Autodesk Fusion 360 part; units mm, degrees
(part 8 of 14)
  line L3484 (76.692, 59.464) -> (76.692, 60.314)
  arc A2247 (75.7545, 60.189) -> (75.6295, 60.189) centre (75.692, 60.189) ccw
  line L3485 (77.242, 58.9765) -> (77.842, 58.9765)
  line L3486 (76.6295, 60.189) -> (76.6295, 59.589)
  line L3487 (76.192, 55.764) -> (76.192, 56.614)
  line L3488 (76.2545, 59.589) -> (76.2545, 60.189)
  line L3489 (75.7545, 59.589) -> (75.7545, 60.189)
  line L3490 (77.967, 58.039) -> (77.117, 58.039)
  line L3491 (76.692, 55.764) -> (76.692, 56.614)
  arc A2248 (75.1295, 59.589) -> (75.2545, 59.589) centre (75.192, 59.589) ccw
  line L3492 (74.692, 59.464) -> (74.692, 60.314)
  line L3493 (76.192, 59.464) -> (76.192, 60.314)
  line L3494 (76.692, 55.764) -> (76.692, 56.614)
  line L3495 (74.142, 59.1015) -> (73.542, 59.1015)
  line L3496 (74.6295, 60.189) -> (74.6295, 59.589)
  arc A2249 (76.6295, 55.889) -> (76.7545, 55.889) centre (76.692, 55.889) ccw
  line L3497 (74.267, 58.539) -> (73.417, 58.539)
  arc A2250 (73.542, 58.6015) -> (73.542, 58.4765) centre (73.542, 58.539) ccw
  arc A2251 (74.142, 57.9765) -> (74.142, 58.1015) centre (74.142, 58.039) ccw
  arc A2252 (80.495, 51.1923) -> (80.495, 51.2558) centre (80.495, 51.224) ccw
  line L3498 (73.542, 56.9765) -> (74.142, 56.9765)
  line L3499 (81.745, 51.782) -> (81.745, 51.224)
  arc A2253 (79.545, 50.9358) -> (79.545, 50.8723) centre (79.545, 50.904) ccw
  line L3500 (79.545, 50.904) -> (80.495, 50.904)
  line L3501 (74.267, 57.539) -> (73.417, 57.539)
  arc A2254 (79.545, 51.8137) -> (79.545, 51.7502) centre (79.545, 51.782) ccw
  line L3502 (79.545, 51.224) -> (79.545, 51.782)
  arc A2255 (74.142, 58.4765) -> (74.142, 58.6015) centre (74.142, 58.539) ccw
  arc A2256 (73.542, 57.6015) -> (73.542, 57.4765) centre (73.542, 57.539) ccw
  line L3503 (73.542, 57.4765) -> (74.142, 57.4765)
  line L3504 (74.142, 57.1015) -> (73.542, 57.1015)
  line L3505 (74.267, 57.039) -> (73.417, 57.039)
  arc A2257 (74.142, 57.4765) -> (74.142, 57.6015) centre (74.142, 57.539) ccw
  line L3506 (78.78, 53.054) -> (78.645, 52.919)
  line L3507 (80.785, 50.904) -> (81.745, 50.904)
  line L3508 (80.785, 51.224) -> (80.785, 52.154)
  arc A2258 (81.745, 50.2943) -> (81.745, 50.3578) centre (81.745, 50.326) ccw
  arc A2259 (80.785, 49.9223) -> (80.785, 49.9858) centre (80.785, 49.954) ccw
  line L3509 (73.542, 57.9765) -> (74.142, 57.9765)
  arc A2260 (80.495, 49.9858) -> (80.495, 49.9223) centre (80.495, 49.954) ccw
  line L3510 (80.495, 52.154) -> (80.495, 51.224)
  line L3511 (80.495, 49.954) -> (79.917, 49.954)
  line L3512 (74.142, 58.1015) -> (73.542, 58.1015)
  arc A2261 (79.545, 51.1923) -> (79.545, 51.2558) centre (79.545, 51.224) ccw
  line L3513 (79.917, 52.154) -> (80.495, 52.154)
  line L3514 (75.692, 56.964) -> (75.692, 59.114)
  line L3515 (81.373, 49.954) -> (80.785, 49.954)
  line L3516 (79.917, 49.954) -> (79.545, 50.326)
  line L3517 (81.745, 50.904) -> (81.745, 50.326)
  arc A2262 (81.373, 49.9223) -> (81.373, 49.9858) centre (81.373, 49.954) ccw
  line L3518 (81.745, 50.326) -> (81.373, 49.954)
  arc A2263 (81.745, 50.8723) -> (81.745, 50.9358) centre (81.745, 50.904) ccw
  arc A2264 (73.542, 58.1015) -> (73.542, 57.9765) centre (73.542, 58.039) ccw
  line L3519 (74.267, 58.039) -> (73.417, 58.039)
  arc A2265 (74.142, 56.9765) -> (74.142, 57.1015) centre (74.142, 57.039) ccw
  line L3520 (74.267, 57.539) -> (73.417, 57.539)
  line L3521 (75.692, 56.964) -> (75.692, 59.114)
  arc A2266 (81.745, 51.2558) -> (81.745, 51.1923) centre (81.745, 51.224) ccw
  arc A2267 (80.785, 49.9858) -> (80.785, 49.9223) centre (80.785, 49.954) ccw
  line L3522 (74.142, 57.6015) -> (73.542, 57.6015)
  line L3523 (81.62, 52.654) -> (81.62, 53.454)
  arc A2268 (80.495, 52.1857) -> (80.495, 52.1222) centre (80.495, 52.154) ccw
  line L3524 (73.542, 58.4765) -> (74.142, 58.4765)
  arc A2269 (81.373, 52.1222) -> (81.373, 52.1857) centre (81.373, 52.154) ccw
  line L3525 (74.267, 58.039) -> (73.417, 58.039)
  arc A2270 (81.745, 50.3578) -> (81.745, 50.2943) centre (81.745, 50.326) ccw
  line L3526 (74.267, 57.039) -> (73.417, 57.039)
  line L3527 (80.495, 50.904) -> (80.495, 49.954)
  arc A2271 (81.373, 52.1857) -> (81.373, 52.1222) centre (81.373, 52.154) ccw
  arc A2272 (79.545, 51.2558) -> (79.545, 51.1923) centre (79.545, 51.224) ccw
  line L3528 (79.545, 50.326) -> (79.545, 50.904)
  arc A2273 (80.785, 50.8723) -> (80.785, 50.9358) centre (80.785, 50.904) ccw
  arc A2274 (79.545, 50.8723) -> (79.545, 50.9358) centre (79.545, 50.904) ccw
  arc A2275 (76.067, 58.039) -> (75.317, 58.039) centre (75.692, 58.039) ccw
  arc A2276 (80.785, 50.9358) -> (80.785, 50.8723) centre (80.785, 50.904) ccw
  arc A2277 (81.373, 49.9858) -> (81.373, 49.9223) centre (81.373, 49.954) ccw
  arc A2278 (73.542, 57.1015) -> (73.542, 56.9765) centre (73.542, 57.039) ccw
  arc A2279 (80.495, 50.8723) -> (80.495, 50.9358) centre (80.495, 50.904) ccw
  arc A2280 (81.745, 50.9358) -> (81.745, 50.8723) centre (81.745, 50.904) ccw
  arc A2281 (75.317, 58.039) -> (76.067, 58.039) centre (75.692, 58.039) ccw
  line L3529 (80.32, 52.654) -> (80.32, 53.454)
  line L3530 (78.645, 52.919) -> (78.645, 49.189)
  line L3531 (81.745, 51.224) -> (80.785, 51.224)
  arc A2282 (80.495, 50.9358) -> (80.495, 50.8723) centre (80.495, 50.904) ccw
  line L3532 (81.62, 52.654) -> (81.62, 53.454)
  line L3533 (78.78, 49.054) -> (82.51, 49.054)
  line L3534 (79.545, 51.782) -> (79.917, 52.154)
  arc A2283 (80.495, 49.9223) -> (80.495, 49.9858) centre (80.495, 49.954) ccw
  line L3535 (79.045, 51.379) -> (78.245, 51.379)
  arc A2284 (82.13, 53.919) -> (82.13, 53.519) centre (82.13, 53.719) ccw
  line L3536 (79.045, 51.379) -> (78.245, 51.379)
  line L3537 (79.045, 52.029) -> (78.245, 52.029)
  line L3538 (79.045, 51.379) -> (78.245, 51.379)
  line L3539 (79.045, 50.079) -> (78.245, 50.079)
  arc A2285 (79.917, 52.1222) -> (79.917, 52.1857) centre (79.917, 52.154) ccw
  line L3540 (79.67, 48.654) -> (79.67, 49.454)
  arc A2286 (79.917, 52.1857) -> (79.917, 52.1222) centre (79.917, 52.154) ccw
  arc A2287 (80.495, 51.2558) -> (80.495, 51.1923) centre (80.495, 51.224) ccw
  line L3541 (80.97, 52.654) -> (80.97, 53.454)
  line L3542 (79.67, 52.654) -> (79.67, 53.454)
  arc A2288 (82.045, 52.754) -> (82.045, 52.354) centre (82.045, 52.554) ccw
  line L3543 (82.51, 53.054) -> (78.78, 53.054)
  arc A2289 (80.785, 52.1857) -> (80.785, 52.1222) centre (80.785, 52.154) ccw
  line L3544 (81.373, 52.154) -> (81.745, 51.782)
  line L3545 (79.045, 50.079) -> (78.245, 50.079)
  line L3546 (79.67, 48.654) -> (79.67, 49.454)
  line L3547 (79.045, 50.729) -> (78.245, 50.729)
  line L3548 (79.67, 52.654) -> (79.67, 53.454)
  arc A2290 (79.545, 50.2943) -> (79.545, 50.3578) centre (79.545, 50.326) ccw
  arc A2291 (79.545, 50.3578) -> (79.545, 50.2943) centre (79.545, 50.326) ccw
  arc A2292 (81.745, 51.8137) -> (81.745, 51.7502) centre (81.745, 51.782) ccw
  arc A2293 (80.785, 51.1923) -> (80.785, 51.2558) centre (80.785, 51.224) ccw
  line L3549 (82.51, 49.054) -> (82.645, 49.189)
  line L3550 (80.97, 48.654) -> (80.97, 49.454)
  arc A2294 (82.13, 53.519) -> (82.13, 53.919) centre (82.13, 53.719) ccw
  line L3551 (79.045, 52.029) -> (78.245, 52.029)
  line L3552 (79.045, 52.029) -> (78.245, 52.029)
  arc A2295 (81.745, 51.1923) -> (81.745, 51.2558) centre (81.745, 51.224) ccw
  line L3553 (81.62, 52.654) -> (81.62, 53.454)
  line L3554 (80.97, 52.654) -> (80.97, 53.454)
  arc A2296 (79.917, 49.9858) -> (79.917, 49.9223) centre (79.917, 49.954) ccw
  line L3555 (80.32, 52.654) -> (80.32, 53.454)
  line L3556 (80.32, 52.654) -> (80.32, 53.454)
  arc A2297 (80.495, 52.1222) -> (80.495, 52.1857) centre (80.495, 52.154) ccw
  arc A2298 (82.045, 52.354) -> (82.045, 52.754) centre (82.045, 52.554) ccw
  line L3557 (82.645, 49.189) -> (82.645, 52.919)
  line L3558 (82.645, 52.919) -> (82.51, 53.054)
  line L3559 (78.645, 49.189) -> (78.78, 49.054)
  line L3560 (79.045, 50.079) -> (78.245, 50.079)
  line L3561 (79.045, 50.729) -> (78.245, 50.729)
  arc A2299 (80.785, 51.2558) -> (80.785, 51.1923) centre (80.785, 51.224) ccw
  line L3562 (80.495, 51.224) -> (79.545, 51.224)
  line L3563 (80.785, 52.154) -> (81.373, 52.154)
  arc A2300 (79.917, 49.9223) -> (79.917, 49.9858) centre (79.917, 49.954) ccw
  line L3564 (79.67, 48.654) -> (79.67, 49.454)
  line L3565 (80.32, 48.654) -> (80.32, 49.454)
  arc A2301 (80.785, 52.1222) -> (80.785, 52.1857) centre (80.785, 52.154) ccw
  arc A2302 (81.745, 51.7502) -> (81.745, 51.8137) centre (81.745, 51.782) ccw
  line L3566 (79.67, 52.654) -> (79.67, 53.454)
  line L3567 (80.97, 52.654) -> (80.97, 53.454)
  line L3568 (80.32, 48.654) -> (80.32, 49.454)
  line L3569 (80.97, 48.654) -> (80.97, 49.454)
  arc A2303 (79.545, 51.7502) -> (79.545, 51.8137) centre (79.545, 51.782) ccw
  line L3570 (80.32, 48.654) -> (80.32, 49.454)
  line L3571 (25.865, 33.063) -> (24.905, 33.063)
  line L3572 (24.905, 33.993) -> (25.493, 33.993)
  arc A2304 (25.493, 34.0247) -> (25.493, 33.9612) centre (25.493, 33.993) ccw
  arc A2305 (24.615, 32.7748) -> (24.615, 32.7113) centre (24.615, 32.743) ccw
  line L3573 (24.615, 33.993) -> (24.615, 33.063)
  arc A2306 (25.865, 33.5892) -> (25.865, 33.6527) centre (25.865, 33.621) ccw
  line L3574 (24.905, 31.793) -> (24.905, 32.743)
  line L3575 (80.6392, 49.71) -> (80.6392, 52.41)
  line L3576 (81.62, 48.654) -> (81.62, 49.454)
  line L3577 (24.615, 31.793) -> (24.037, 31.793)
  arc A2307 (24.615, 31.8248) -> (24.615, 31.7613) centre (24.615, 31.793) ccw
  line L3578 (26.63, 30.893) -> (26.765, 31.028)
  line L3579 (79.045, 50.729) -> (78.245, 50.729)
  line L3580 (25.493, 31.793) -> (24.905, 31.793)
  line L3581 (22.9, 30.893) -> (26.63, 30.893)
  arc A2308 (25.865, 32.7748) -> (25.865, 32.7113) centre (25.865, 32.743) ccw
  line L3582 (83.045, 52.029) -> (82.245, 52.029)
  line L3583 (83.045, 50.079) -> (82.245, 50.079)
  line L3584 (83.045, 51.379) -> (82.245, 51.379)
  line L3585 (83.045, 51.379) -> (82.245, 51.379)
  line L3586 (24.905, 32.743) -> (25.865, 32.743)
  arc A2309 (24.905, 31.8248) -> (24.905, 31.7613) centre (24.905, 31.793) ccw
  line L3587 (24.037, 31.793) -> (23.665, 32.165)
  arc A2310 (24.905, 31.7613) -> (24.905, 31.8248) centre (24.905, 31.793) ccw
  arc A2311 (24.037, 31.8248) -> (24.037, 31.7613) centre (24.037, 31.793) ccw
  line L3588 (25.493, 33.993) -> (25.865, 33.621)
  arc A2312 (24.037, 31.7613) -> (24.037, 31.8248) centre (24.037, 31.793) ccw
  line L3589 (23.665, 33.621) -> (24.037, 33.993)
  arc A2313 (24.615, 31.7613) -> (24.615, 31.8248) centre (24.615, 31.793) ccw
  arc A2314 (24.615, 34.0247) -> (24.615, 33.9612) centre (24.615, 33.993) ccw
  arc A2315 (23.665, 33.0948) -> (23.665, 33.0313) centre (23.665, 33.063) ccw
  arc A2316 (25.865, 32.1333) -> (25.865, 32.1968) centre (25.865, 32.165) ccw
  line L3590 (83.045, 52.029) -> (82.245, 52.029)
  line L3591 (26.63, 34.893) -> (22.9, 34.893)
  arc A2317 (25.493, 31.8248) -> (25.493, 31.7613) centre (25.493, 31.793) ccw
  line L3592 (22.765, 34.758) -> (22.765, 31.028)
  arc A2318 (23.665, 32.1333) -> (23.665, 32.1968) centre (23.665, 32.165) ccw
  line L3593 (83.045, 50.729) -> (82.245, 50.729)
  line L3594 (23.665, 33.063) -> (23.665, 33.621)
  arc A2319 (25.493, 31.7613) -> (25.493, 31.8248) centre (25.493, 31.793) ccw
  line L3595 (25.865, 32.743) -> (25.865, 32.165)
  line L3596 (83.045, 52.029) -> (82.245, 52.029)
  line L3597 (83.045, 50.079) -> (82.245, 50.079)
  line L3598 (80.6392, 49.71) -> (80.6392, 52.41)
  line L3599 (25.865, 32.165) -> (25.493, 31.793)
  line L3600 (23.665, 32.743) -> (24.615, 32.743)
  line L3601 (83.045, 50.729) -> (82.245, 50.729)
  line L3602 (23.665, 32.165) -> (23.665, 32.743)
  arc A2320 (24.905, 32.7113) -> (24.905, 32.7748) centre (24.905, 32.743) ccw
  line L3603 (24.615, 32.743) -> (24.615, 31.793)
  line L3604 (81.62, 48.654) -> (81.62, 49.454)
  line L3605 (83.045, 51.379) -> (82.245, 51.379)
  line L3606 (83.045, 50.079) -> (82.245, 50.079)
  arc A2321 (25.865, 32.1968) -> (25.865, 32.1333) centre (25.865, 32.165) ccw
  arc A2322 (25.865, 32.7113) -> (25.865, 32.7748) centre (25.865, 32.743) ccw
  line L3607 (83.045, 50.729) -> (82.245, 50.729)
  line L3608 (80.97, 48.654) -> (80.97, 49.454)
  line L3609 (81.62, 48.654) -> (81.62, 49.454)
  arc A2323 (24.905, 33.0313) -> (24.905, 33.0948) centre (24.905, 33.063) ccw
  line L3610 (25.865, 33.621) -> (25.865, 33.063)
  arc A2324 (24.037, 33.9612) -> (24.037, 34.0247) centre (24.037, 33.993) ccw
  arc A2325 (24.905, 32.7748) -> (24.905, 32.7113) centre (24.905, 32.743) ccw
  line L3611 (26.765, 34.758) -> (26.63, 34.893)
  line L3612 (22.765, 31.028) -> (22.9, 30.893)
  line L3613 (24.44, 30.493) -> (24.44, 31.293)
  arc A2326 (26.165, 34.193) -> (26.165, 34.593) centre (26.165, 34.393) ccw
  line L3614 (24.44, 30.493) -> (24.44, 31.293)
  line L3615 (24.037, 33.993) -> (24.615, 33.993)
  arc A2327 (25.493, 33.9612) -> (25.493, 34.0247) centre (25.493, 33.993) ccw
  arc A2328 (24.905, 34.0247) -> (24.905, 33.9612) centre (24.905, 33.993) ccw
  line L3616 (23.79, 34.493) -> (23.79, 35.293)
  line L3617 (23.165, 33.218) -> (22.365, 33.218)
  arc A2329 (23.665, 32.1968) -> (23.665, 32.1333) centre (23.665, 32.165) ccw
  line L3618 (23.165, 32.568) -> (22.365, 32.568)
  arc A2330 (23.665, 32.7748) -> (23.665, 32.7113) centre (23.665, 32.743) ccw
  line L3619 (25.09, 30.493) -> (25.09, 31.293)
  line L3620 (29.684, 53.256) -> (29.106, 53.256)
  line L3621 (27.165, 31.918) -> (26.365, 31.918)
  line L3622 (24.615, 33.063) -> (23.665, 33.063)
  line L3623 (23.79, 34.493) -> (23.79, 35.293)
  arc A2331 (26.25, 35.758) -> (26.25, 35.358) centre (26.25, 35.558) ccw
  line L3624 (23.165, 31.918) -> (22.365, 31.918)
  line L3625 (23.165, 33.868) -> (22.365, 33.868)
  arc A2332 (24.615, 33.0313) -> (24.615, 33.0948) centre (24.615, 33.063) ccw
  line L3626 (25.09, 34.493) -> (25.09, 35.293)
  arc A2333 (23.665, 33.0313) -> (23.665, 33.0948) centre (23.665, 33.063) ccw
  arc A2334 (24.615, 33.9612) -> (24.615, 34.0247) centre (24.615, 33.993) ccw
  line L3627 (23.165, 32.568) -> (22.365, 32.568)
  line L3628 (23.165, 33.218) -> (22.365, 33.218)
  line L3629 (29.106, 53.256) -> (29.106, 54.206)
  arc A2335 (24.037, 34.0247) -> (24.037, 33.9612) centre (24.037, 33.993) ccw
  line L3630 (29.106, 54.206) -> (30.056, 54.206)
  line L3631 (23.79, 30.493) -> (23.79, 31.293)
  arc A2336 (23.665, 32.7113) -> (23.665, 32.7748) centre (23.665, 32.743) ccw
  line L3632 (25.74, 34.493) -> (25.74, 35.293)
  line L3633 (25.09, 30.493) -> (25.09, 31.293)
  arc A2337 (23.665, 33.5892) -> (23.665, 33.6527) centre (23.665, 33.621) ccw
  line L3634 (30.056, 54.206) -> (30.056, 53.628)
  line L3635 (25.74, 34.493) -> (25.74, 35.293)
  line L3636 (23.165, 33.868) -> (22.365, 33.868)
  line L3637 (24.44, 34.493) -> (24.44, 35.293)
  line L3638 (26.765, 31.028) -> (26.765, 34.758)
  line L3639 (25.74, 34.493) -> (25.74, 35.293)
  line L3640 (24.905, 33.063) -> (24.905, 33.993)
  line L3641 (25.09, 34.493) -> (25.09, 35.293)
  arc A2338 (24.905, 33.9612) -> (24.905, 34.0247) centre (24.905, 33.993) ccw
  line L3642 (23.165, 33.218) -> (22.365, 33.218)
  arc A2339 (24.615, 32.7113) -> (24.615, 32.7748) centre (24.615, 32.743) ccw
  arc A2340 (24.615, 33.0948) -> (24.615, 33.0313) centre (24.615, 33.063) ccw
  line L3643 (24.44, 30.493) -> (24.44, 31.293)
  line L3644 (22.9, 34.893) -> (22.765, 34.758)
  arc A2341 (25.865, 33.0313) -> (25.865, 33.0948) centre (25.865, 33.063) ccw
  arc A2342 (25.865, 33.0948) -> (25.865, 33.0313) centre (25.865, 33.063) ccw
  line L3645 (23.79, 30.493) -> (23.79, 31.293)
  line L3646 (23.79, 30.493) -> (23.79, 31.293)
  arc A2343 (25.865, 33.6527) -> (25.865, 33.5892) centre (25.865, 33.621) ccw
  arc A2344 (24.905, 33.0948) -> (24.905, 33.0313) centre (24.905, 33.063) ccw
  arc A2345 (26.25, 35.358) -> (26.25, 35.758) centre (26.25, 35.558) ccw
  line L3647 (23.165, 33.868) -> (22.365, 33.868)
  line L3648 (23.79, 34.493) -> (23.79, 35.293)
  line L3649 (24.44, 34.493) -> (24.44, 35.293)
  arc A2346 (23.665, 33.6527) -> (23.665, 33.5892) centre (23.665, 33.621) ccw
  line L3650 (23.165, 31.918) -> (22.365, 31.918)
  line L3651 (23.165, 31.918) -> (22.365, 31.918)
  line L3652 (23.165, 32.568) -> (22.365, 32.568)
  line L3653 (25.09, 34.493) -> (25.09, 35.293)
  arc A2347 (26.165, 34.593) -> (26.165, 34.193) centre (26.165, 34.393) ccw
  line L3654 (24.44, 34.493) -> (24.44, 35.293)
  line L3655 (27.165, 33.218) -> (26.365, 33.218)
  line L3656 (28.228, 55.456) -> (28.786, 55.456)
  arc A2348 (29.1377, 54.496) -> (29.0742, 54.496) centre (29.106, 54.496) ccw
  arc A2349 (28.1963, 53.256) -> (28.2598, 53.256) centre (28.228, 53.256) ccw
  arc A2350 (30.0242, 55.084) -> (30.0877, 55.084) centre (30.056, 55.084) ccw
  arc A2351 (28.7542, 53.256) -> (28.8177, 53.256) centre (28.786, 53.256) ccw
  arc A2352 (29.7157, 53.256) -> (29.6522, 53.256) centre (29.684, 53.256) ccw
  arc A2353 (30.0877, 53.628) -> (30.0242, 53.628) centre (30.056, 53.628) ccw
  arc A2354 (30.0242, 54.206) -> (30.0877, 54.206) centre (30.056, 54.206) ccw
  arc A2355 (28.2598, 53.256) -> (28.1963, 53.256) centre (28.228, 53.256) ccw
  line L3657 (27.356, 55.331) -> (26.556, 55.331)
  arc A2356 (30.0877, 54.496) -> (30.0242, 54.496) centre (30.056, 54.496) ccw
  arc A2357 (29.0742, 55.456) -> (29.1377, 55.456) centre (29.106, 55.456) ccw
  line L3658 (27.165, 33.218) -> (26.365, 33.218)
  line L3659 (27.165, 33.868) -> (26.365, 33.868)
  line L3660 (27.356, 54.681) -> (26.556, 54.681)
  line L3661 (27.091, 52.356) -> (30.821, 52.356)
  line L3662 (27.856, 53.628) -> (27.856, 54.206)
  arc A2358 (27.8878, 54.496) -> (27.8243, 54.496) centre (27.856, 54.496) ccw
  arc A2359 (26.091, 55.841) -> (26.491, 55.841) centre (26.291, 55.841) ccw
  line L3663 (25.74, 30.493) -> (25.74, 31.293)
  line L3664 (29.106, 55.456) -> (29.684, 55.456)
  line L3665 (27.856, 55.084) -> (28.228, 55.456)
  line L3666 (26.956, 52.491) -> (27.091, 52.356)
  line L3667 (27.856, 54.206) -> (28.786, 54.206)
  line L3668 (27.856, 54.496) -> (27.856, 55.084)
  arc A2360 (29.6522, 55.456) -> (29.7157, 55.456) centre (29.684, 55.456) ccw
  line L3669 (27.356, 55.331) -> (26.556, 55.331)
  arc A2361 (27.8878, 53.628) -> (27.8243, 53.628) centre (27.856, 53.628) ccw
  arc A2362 (30.0877, 55.084) -> (30.0242, 55.084) centre (30.056, 55.084) ccw
  line L3670 (29.684, 55.456) -> (30.056, 55.084)
  line L3671 (25.74, 30.493) -> (25.74, 31.293)
  line L3672 (30.056, 55.084) -> (30.056, 54.496)
  line L3673 (25.09, 30.493) -> (25.09, 31.293)
  line L3674 (27.165, 32.568) -> (26.365, 32.568)
  arc A2363 (28.8177, 53.256) -> (28.7542, 53.256) centre (28.786, 53.256) ccw
  line L3675 (27.165, 32.568) -> (26.365, 32.568)
  arc A2364 (29.0742, 54.496) -> (29.1377, 54.496) centre (29.106, 54.496) ccw
  line L3676 (25.74, 30.493) -> (25.74, 31.293)
  line L3677 (27.165, 31.918) -> (26.365, 31.918)
  line L3678 (27.165, 32.568) -> (26.365, 32.568)
  line L3679 (28.786, 54.206) -> (28.786, 53.256)
  line L3680 (27.165, 33.868) -> (26.365, 33.868)
  line L3681 (27.165, 33.218) -> (26.365, 33.218)
  line L3682 (30.956, 52.491) -> (30.956, 56.221)
  arc A2365 (30.0242, 53.628) -> (30.0877, 53.628) centre (30.056, 53.628) ccw
  line L3683 (24.7592, 31.549) -> (24.7592, 34.249)
  arc A2366 (27.8878, 54.206) -> (27.8243, 54.206) centre (27.856, 54.206) ccw
  arc A2367 (29.0742, 53.256) -> (29.1377, 53.256) centre (29.106, 53.256) ccw
  line L3684 (30.056, 53.628) -> (29.684, 53.256)
  arc A2368 (29.7157, 55.456) -> (29.6522, 55.456) centre (29.684, 55.456) ccw
  arc A2369 (28.7542, 54.206) -> (28.8177, 54.206) centre (28.786, 54.206) ccw
  arc A2370 (30.0877, 54.206) -> (30.0242, 54.206) centre (30.056, 54.206) ccw
  line L3685 (27.091, 56.356) -> (26.956, 56.221)
  arc A2371 (30.0242, 54.496) -> (30.0877, 54.496) centre (30.056, 54.496) ccw
  arc A2372 (29.1377, 55.456) -> (29.0742, 55.456) centre (29.106, 55.456) ccw
  arc A2373 (28.7542, 55.456) -> (28.8177, 55.456) centre (28.786, 55.456) ccw
  line L3686 (27.165, 33.868) -> (26.365, 33.868)
  line L3687 (24.7592, 31.549) -> (24.7592, 34.249)
  line L3688 (27.165, 31.918) -> (26.365, 31.918)
  line L3689 (30.821, 56.356) -> (27.091, 56.356)
  line L3690 (30.956, 56.221) -> (30.821, 56.356)
  line L3691 (30.056, 54.496) -> (29.106, 54.496)
  line L3692 (29.106, 54.496) -> (29.106, 55.456)
  line L3693 (26.956, 56.221) -> (26.956, 52.491)
  line L3694 (27.356, 54.681) -> (26.556, 54.681)
  line L3695 (27.356, 55.331) -> (26.556, 55.331)
  line L3696 (31.356, 54.031) -> (30.556, 54.031)
  line L3697 (28.631, 52.756) -> (28.631, 51.956)
  line L3698 (29.931, 56.756) -> (29.931, 55.956)
  line L3699 (29.931, 52.756) -> (29.931, 51.956)
  line L3700 (27.356, 53.381) -> (26.556, 53.381)
  line L3701 (27.356, 54.681) -> (26.556, 54.681)
  line L3702 (36.495, 52.97) -> (37.495, 53.97)
  line L3703 (57.795, 52.97) -> (57.795, 46.73)
  line L3704 (28.228, 53.256) -> (27.856, 53.628)
  arc A2374 (27.8878, 55.084) -> (27.8243, 55.084) centre (27.856, 55.084) ccw
  arc A2375 (28.7542, 54.496) -> (28.8177, 54.496) centre (28.786, 54.496) ccw
  line L3705 (28.631, 52.756) -> (28.631, 51.956)
  line L3706 (29.281, 52.756) -> (29.281, 51.956)
  line L3707 (31.356, 53.381) -> (30.556, 53.381)
  line L3708 (37.455, 46.88) -> (37.965, 48.22)
  line L3709 (39.895, 46.3495) -> (39.895, 48.6225)
  line L3710 (31.356, 53.381) -> (30.556, 53.381)
  line L3711 (28.786, 55.456) -> (28.786, 54.496)
  arc A2376 (27.8243, 55.084) -> (27.8878, 55.084) centre (27.856, 55.084) ccw
  line L3712 (28.631, 56.756) -> (28.631, 55.956)
  line L3713 (27.981, 56.756) -> (27.981, 55.956)
  arc A2377 (36.195, 53.01) -> (37.995, 53.01) centre (37.095, 53.01) ccw
  line L3714 (56.795, 53.97) -> (57.795, 52.97)
  arc A2378 (27.256, 55.756) -> (27.656, 55.756) centre (27.456, 55.756) ccw
  line L3715 (36.495, 46.73) -> (36.495, 52.97)
  line L3716 (31.356, 53.381) -> (30.556, 53.381)
  arc A2379 (28.8177, 55.456) -> (28.7542, 55.456) centre (28.786, 55.456) ccw
  arc A2380 (28.1963, 55.456) -> (28.2598, 55.456) centre (28.228, 55.456) ccw
  line L3717 (28.786, 53.256) -> (28.228, 53.256)
  line L3718 (27.356, 53.381) -> (26.556, 53.381)
  line L3719 (30.821, 52.356) -> (30.956, 52.491)
  arc A2381 (27.8243, 54.206) -> (27.8878, 54.206) centre (27.856, 54.206) ccw
  line L3720 (27.981, 52.756) -> (27.981, 51.956)
  arc A2382 (28.8177, 54.496) -> (28.7542, 54.496) centre (28.786, 54.496) ccw
  arc A2383 (29.1377, 54.206) -> (29.0742, 54.206) centre (29.106, 54.206) ccw
  line L3721 (27.356, 54.031) -> (26.556, 54.031)
  line L3722 (27.981, 52.756) -> (27.981, 51.956)
  line L3723 (29.931, 52.756) -> (29.931, 51.956)
  line L3724 (31.356, 54.031) -> (30.556, 54.031)
  arc A2384 (28.8177, 54.206) -> (28.7542, 54.206) centre (28.786, 54.206) ccw
  arc A2385 (29.0742, 54.206) -> (29.1377, 54.206) centre (29.106, 54.206) ccw
  line L3725 (29.281, 52.756) -> (29.281, 51.956)
  line L3726 (28.631, 52.756) -> (28.631, 51.956)
  line L3727 (31.356, 54.681) -> (30.556, 54.681)
  line L3728 (31.356, 54.681) -> (30.556, 54.681)
  line L3729 (27.981, 52.756) -> (27.981, 51.956)
  arc A2386 (28.2598, 55.456) -> (28.1963, 55.456) centre (28.228, 55.456) ccw
  arc A2387 (29.1377, 53.256) -> (29.0742, 53.256) centre (29.106, 53.256) ccw
  line L3730 (27.356, 54.031) -> (26.556, 54.031)
  line L3731 (29.281, 52.756) -> (29.281, 51.956)
  line L3732 (29.931, 56.756) -> (29.931, 55.956)
  arc A2388 (27.8243, 53.628) -> (27.8878, 53.628) centre (27.856, 53.628) ccw
  arc A2389 (27.656, 55.756) -> (27.256, 55.756) centre (27.456, 55.756) ccw
  line L3733 (31.356, 54.031) -> (30.556, 54.031)
  arc A2390 (27.8243, 54.496) -> (27.8878, 54.496) centre (27.856, 54.496) ccw
  line L3734 (28.786, 54.496) -> (27.856, 54.496)
  line L3735 (27.356, 53.381) -> (26.556, 53.381)
  line L3736 (29.931, 52.756) -> (29.931, 51.956)
  line L3737 (27.356, 54.031) -> (26.556, 54.031)
  arc A2391 (29.6522, 53.256) -> (29.7157, 53.256) centre (29.684, 53.256) ccw
  arc A2392 (26.491, 55.841) -> (26.091, 55.841) centre (26.291, 55.841) ccw
  line L3738 (42.395, 46.3495) -> (42.395, 48.6225)
  line L3739 (42.895, 46.3495) -> (42.895, 48.6225)
  line L3740 (42.395, 52.0775) -> (42.395, 54.3505)
  line L3741 (41.395, 52.0775) -> (41.395, 54.3505)
  line L3742 (42.895, 46.3495) -> (42.895, 48.6225)
  line L3743 (43.395, 46.3495) -> (43.395, 48.6225)
  line L3744 (39.895, 46.3495) -> (39.895, 48.6225)
  line L3745 (40.895, 46.3495) -> (40.895, 48.6225)
  line L3746 (40.395, 46.3495) -> (40.395, 48.6225)
  line L3747 (42.395, 52.0775) -> (42.395, 54.3505)
  line L3748 (31.356, 55.331) -> (30.556, 55.331)
  line L3749 (31.356, 55.331) -> (30.556, 55.331)
  arc A2393 (37.995, 53.01) -> (36.195, 53.01) centre (37.095, 53.01) ccw
  line L3750 (39.895, 52.0775) -> (39.895, 54.3505)
  line L3751 (28.631, 56.756) -> (28.631, 55.956)
  line L3752 (27.981, 56.756) -> (27.981, 55.956)
  line L3753 (31.356, 54.681) -> (30.556, 54.681)
  line L3754 (41.395, 52.0775) -> (41.395, 54.3505)
  line L3755 (31.356, 55.331) -> (30.556, 55.331)
  line L3756 (41.395, 46.3495) -> (41.395, 48.6225)
  line L3757 (40.395, 46.3495) -> (40.395, 48.6225)
  line L3758 (39.895, 52.0775) -> (39.895, 54.3505)
  line L3759 (29.281, 56.756) -> (29.281, 55.956)
  line L3760 (41.895, 46.3495) -> (41.895, 48.6225)
  line L3761 (39.895, 52.0775) -> (39.895, 54.3505)
  line L3762 (41.895, 46.3495) -> (41.895, 48.6225)
  line L3763 (44.395, 46.3495) -> (44.395, 48.6225)
  line L3764 (43.395, 46.3495) -> (43.395, 48.6225)
  line L3765 (37.965, 48.22) -> (38.445, 46.86)
  line L3766 (28.631, 56.756) -> (28.631, 55.956)
  line L3767 (41.395, 46.3495) -> (41.395, 48.6225)
  line L3768 (40.895, 46.3495) -> (40.895, 48.6225)
  line L3769 (40.895, 52.0775) -> (40.895, 54.3505)
  line L3770 (42.895, 46.3495) -> (42.895, 48.6225)
  line L3771 (42.895, 52.0775) -> (42.895, 54.3505)
  line L3772 (30.3, 54.3502) -> (27.6, 54.3502)
  arc A2394 (58.085, 53.01) -> (56.285, 53.01) centre (57.185, 53.01) ccw
  line L3773 (40.395, 46.3495) -> (40.395, 48.6225)
  line L3774 (29.281, 56.756) -> (29.281, 55.956)
  line L3775 (30.3, 54.3502) -> (27.6, 54.3502)
  line L3776 (57.795, 46.73) -> (36.495, 46.73)
  line L3777 (39.895, 46.3495) -> (39.895, 48.6225)
  line L3778 (41.395, 52.0775) -> (41.395, 54.3505)
  line L3779 (29.281, 56.756) -> (29.281, 55.956)
  line L3780 (40.895, 46.3495) -> (40.895, 48.6225)
  line L3781 (41.895, 52.0775) -> (41.895, 54.3505)
  line L3782 (40.395, 52.0775) -> (40.395, 54.3505)
  line L3783 (40.895, 52.0775) -> (40.895, 54.3505)
  line L3784 (40.395, 52.0775) -> (40.395, 54.3505)
  line L3785 (41.895, 52.0775) -> (41.895, 54.3505)
  line L3786 (42.395, 46.3495) -> (42.395, 48.6225)
  line L3787 (43.395, 52.0775) -> (43.395, 54.3505)
  arc A2395 (56.285, 53.01) -> (58.085, 53.01) centre (57.185, 53.01) ccw
  line L3788 (41.895, 52.0775) -> (41.895, 54.3505)
  line L3789 (41.395, 46.3495) -> (41.395, 48.6225)
  line L3790 (27.981, 56.756) -> (27.981, 55.956)
  line L3791 (40.395, 52.0775) -> (40.395, 54.3505)
  line L3792 (29.931, 56.756) -> (29.931, 55.956)
  line L3793 (44.395, 46.3495) -> (44.395, 48.6225)
  line L3794 (40.895, 52.0775) -> (40.895, 54.3505)
  line L3795 (37.495, 53.97) -> (56.795, 53.97)
  line L3796 (43.895, 52.0775) -> (43.895, 54.3505)
  line L3797 (41.895, 46.3495) -> (41.895, 48.6225)
  line L3798 (42.895, 52.0775) -> (42.895, 54.3505)
  line L3799 (61.3283, 55.598) -> (60.4393, 55.598)
  line L3800 (61.623, 55.8927) -> (61.623, 56.7817)
  line L3801 (64.623, 55.8927) -> (64.623, 56.7817)
  line L3802 (63.123, 55.8927) -> (63.123, 56.7817)
  line L3803 (43.895, 46.3495) -> (43.895, 48.6225)
  line L3804 (45.395, 52.0775) -> (45.395, 54.3505)
  line L3805 (44.895, 46.3495) -> (44.895, 48.6225)
  line L3806 (61.3283, 55.098) -> (60.4393, 55.098)
  line L3807 (62.123, 55.8927) -> (62.123, 56.7817)
  line L3808 (61.3283, 55.598) -> (60.4393, 55.598)
  line L3809 (43.895, 52.0775) -> (43.895, 54.3505)
  line L3810 (63.623, 55.8927) -> (63.623, 56.7817)
  line L3811 (43.895, 46.3495) -> (43.895, 48.6225)
  line L3812 (46.395, 46.3495) -> (46.395, 48.6225)
  line L3813 (63.123, 55.8927) -> (63.123, 56.7817)
  line L3814 (45.395, 46.3495) -> (45.395, 48.6225)
  line L3815 (43.395, 52.0775) -> (43.395, 54.3505)
  line L3816 (45.395, 52.0775) -> (45.395, 54.3505)
  line L3817 (44.395, 52.0775) -> (44.395, 54.3505)
  line L3818 (63.623, 55.8927) -> (63.623, 56.7817)
  line L3819 (62.623, 55.8927) -> (62.623, 56.7817)
  line L3820 (44.395, 52.0775) -> (44.395, 54.3505)
  line L3821 (44.895, 46.3495) -> (44.895, 48.6225)
  line L3822 (61.3283, 55.598) -> (60.4393, 55.598)
  line L3823 (64.123, 55.8927) -> (64.123, 56.7817)
  line L3824 (48.895, 52.0775) -> (48.895, 54.3505)
  line L3825 (62.623, 55.8927) -> (62.623, 56.7817)
  line L3826 (49.895, 46.3495) -> (49.895, 48.6225)
  line L3827 (62.123, 55.8927) -> (62.123, 56.7817)
  line L3828 (63.623, 55.8927) -> (63.623, 56.7817)
  line L3829 (44.895, 52.0775) -> (44.895, 54.3505)
  line L3830 (62.623, 55.8927) -> (62.623, 56.7817)
  line L3831 (61.623, 55.8927) -> (61.623, 56.7817)
  line L3832 (44.895, 52.0775) -> (44.895, 54.3505)
  line L3833 (65.123, 55.8927) -> (65.123, 56.7817)
  line L3834 (43.895, 52.0775) -> (43.895, 54.3505)
  line L3835 (44.895, 52.0775) -> (44.895, 54.3505)
  line L3836 (42.395, 52.0775) -> (42.395, 54.3505)
  line L3837 (64.123, 55.8927) -> (64.123, 56.7817)
  line L3838 (43.895, 46.3495) -> (43.895, 48.6225)
  line L3839 (45.895, 46.3495) -> (45.895, 48.6225)
  line L3840 (45.395, 46.3495) -> (45.395, 48.6225)
  line L3841 (45.895, 46.3495) -> (45.895, 48.6225)
  line L3842 (44.395, 46.3495) -> (44.395, 48.6225)
  line L3843 (43.395, 52.0775) -> (43.395, 54.3505)
  line L3844 (44.395, 52.0775) -> (44.395, 54.3505)
  line L3845 (42.895, 52.0775) -> (42.895, 54.3505)
  line L3846 (45.395, 46.3495) -> (45.395, 48.6225)
  line L3847 (44.895, 46.3495) -> (44.895, 48.6225)
  line L3848 (45.895, 52.0775) -> (45.895, 54.3505)
  line L3849 (45.895, 52.0775) -> (45.895, 54.3505)
  line L3850 (43.395, 46.3495) -> (43.395, 48.6225)
  line L3851 (45.895, 46.3495) -> (45.895, 48.6225)
  line L3852 (45.895, 52.0775) -> (45.895, 54.3505)
  line L3853 (62.123, 55.8927) -> (62.123, 56.7817)
  line L3854 (64.123, 55.8927) -> (64.123, 56.7817)
  line L3855 (45.395, 52.0775) -> (45.395, 54.3505)
  line L3856 (61.3283, 55.098) -> (60.4393, 55.098)
  line L3857 (64.623, 55.8927) -> (64.623, 56.7817)
  line L3858 (65.123, 55.8927) -> (65.123, 56.7817)
  line L3859 (61.623, 55.8927) -> (61.623, 56.7817)
  line L3860 (63.123, 55.8927) -> (63.123, 56.7817)
  line L3861 (42.395, 46.3495) -> (42.395, 48.6225)
  line L3862 (64.623, 55.8927) -> (64.623, 56.7817)
  line L3863 (50.895, 52.0775) -> (50.895, 54.3505)
  line L3864 (53.895, 46.3495) -> (53.895, 48.6225)
  line L3865 (53.895, 52.0775) -> (53.895, 54.3505)
  line L3866 (53.395, 46.3495) -> (53.395, 48.6225)
  line L3867 (54.395, 46.3495) -> (54.395, 48.6225)
  line L3868 (53.395, 46.3495) -> (53.395, 48.6225)
  line L3869 (49.395, 46.3495) -> (49.395, 48.6225)
  line L3870 (50.395, 52.0775) -> (50.395, 54.3505)
  line L3871 (52.395, 46.3495) -> (52.395, 48.6225)
  line L3872 (51.395, 52.0775) -> (51.395, 54.3505)
  line L3873 (53.895, 52.0775) -> (53.895, 54.3505)
  line L3874 (54.395, 52.0775) -> (54.395, 54.3505)
  line L3875 (48.895, 46.3495) -> (48.895, 48.6225)
  line L3876 (51.895, 46.3495) -> (51.895, 48.6225)
  line L3877 (53.895, 52.0775) -> (53.895, 54.3505)
  line L3878 (49.895, 52.0775) -> (49.895, 54.3505)
  line L3879 (49.395, 46.3495) -> (49.395, 48.6225)
  line L3880 (50.895, 46.3495) -> (50.895, 48.6225)
  line L3881 (50.395, 52.0775) -> (50.395, 54.3505)
  line L3882 (49.895, 46.3495) -> (49.895, 48.6225)
  line L3883 (48.895, 52.0775) -> (48.895, 54.3505)
  line L3884 (50.395, 46.3495) -> (50.395, 48.6225)
  line L3885 (50.895, 46.3495) -> (50.895, 48.6225)
  line L3886 (51.395, 52.0775) -> (51.395, 54.3505)
  line L3887 (51.395, 46.3495) -> (51.395, 48.6225)
  line L3888 (52.395, 52.0775) -> (52.395, 54.3505)
  line L3889 (50.895, 52.0775) -> (50.895, 54.3505)
  line L3890 (51.395, 46.3495) -> (51.395, 48.6225)
  line L3891 (52.895, 46.3495) -> (52.895, 48.6225)
  line L3892 (52.895, 52.0775) -> (52.895, 54.3505)
  line L3893 (48.895, 46.3495) -> (48.895, 48.6225)
  line L3894 (49.895, 46.3495) -> (49.895, 48.6225)
  line L3895 (53.395, 52.0775) -> (53.395, 54.3505)
  line L3896 (52.895, 52.0775) -> (52.895, 54.3505)
  line L3897 (51.895, 46.3495) -> (51.895, 48.6225)
  line L3898 (50.395, 46.3495) -> (50.395, 48.6225)
  line L3899 (36.828, 53.016) -> (37.336, 53.016)
  line L3900 (54.395, 52.0775) -> (54.395, 54.3505)
  line L3901 (54.395, 46.3495) -> (54.395, 48.6225)
  line L3902 (49.395, 52.0775) -> (49.395, 54.3505)
  line L3903 (48.895, 52.0775) -> (48.895, 54.3505)
  line L3904 (49.895, 52.0775) -> (49.895, 54.3505)
  line L3905 (51.895, 52.0775) -> (51.895, 54.3505)
  line L3906 (50.395, 52.0775) -> (50.395, 54.3505)
  line L3907 (50.395, 46.3495) -> (50.395, 48.6225)
  line L3908 (49.395, 52.0775) -> (49.395, 54.3505)
  line L3909 (49.395, 46.3495) -> (49.395, 48.6225)
  line L3910 (49.395, 52.0775) -> (49.395, 54.3505)
  line L3911 (51.895, 46.3495) -> (51.895, 48.6225)
  line L3912 (51.395, 46.3495) -> (51.395, 48.6225)
  line L3913 (51.895, 52.0775) -> (51.895, 54.3505)
  line L3914 (48.895, 46.3495) -> (48.895, 48.6225)
  line L3915 (51.395, 52.0775) -> (51.395, 54.3505)
  line L3916 (52.395, 46.3495) -> (52.395, 48.6225)
  line L3917 (52.395, 52.0775) -> (52.395, 54.3505)
  line L3918 (50.895, 46.3495) -> (50.895, 48.6225)
  line L3919 (50.895, 52.0775) -> (50.895, 54.3505)
  line L3920 (52.395, 52.0775) -> (52.395, 54.3505)
  line L3921 (52.895, 46.3495) -> (52.895, 48.6225)
  line L3922 (49.895, 52.0775) -> (49.895, 54.3505)
  line L3923 (52.895, 46.3495) -> (52.895, 48.6225)
  line L3924 (51.895, 52.0775) -> (51.895, 54.3505)
  line L3925 (52.895, 52.0775) -> (52.895, 54.3505)
  line L3926 (52.395, 46.3495) -> (52.395, 48.6225)
  arc A2396 (37.082, 53.3335) -> (37.082, 52.6985) centre (37.082, 53.016) ccw
  line L3927 (37.082, 52.762) -> (37.082, 53.27)
  line L3928 (36.828, 53.016) -> (37.336, 53.016)
  line L3929 (57.208, 52.762) -> (57.208, 53.27)
  arc A2397 (37.336, 53.016) -> (36.828, 53.016) centre (37.082, 53.016) ccw
  arc A2398 (37.336, 53.016) -> (36.828, 53.016) centre (37.082, 53.016) ccw
  arc A2399 (36.828, 53.016) -> (37.336, 53.016) centre (37.082, 53.016) ccw
  line L3930 (37.082, 52.762) -> (37.082, 53.27)
  arc A2400 (57.462, 53.016) -> (56.954, 53.016) centre (57.208, 53.016) ccw
  line L3931 (37.082, 52.762) -> (37.082, 53.27)
  arc A2401 (37.336, 53.016) -> (36.828, 53.016) centre (37.082, 53.016) ccw
  line L3932 (36.828, 53.016) -> (37.336, 53.016)
  line L3933 (53.395, 52.0775) -> (53.395, 54.3505)
  line L3934 (37.082, 52.762) -> (37.082, 53.27)
  line L3935 (37.082, 52.762) -> (37.082, 53.27)
  arc A2402 (37.336, 53.016) -> (36.828, 53.016) centre (37.082, 53.016) ccw
  arc A2403 (36.828, 53.016) -> (37.336, 53.016) centre (37.082, 53.016) ccw
  arc A2404 (37.336, 53.016) -> (36.828, 53.016) centre (37.082, 53.016) ccw
  arc A2405 (36.828, 53.016) -> (37.336, 53.016) centre (37.082, 53.016) ccw
  line L3936 (53.895, 46.3495) -> (53.895, 48.6225)
  arc A2406 (57.462, 53.016) -> (56.954, 53.016) centre (57.208, 53.016) ccw
  arc A2407 (56.954, 53.016) -> (57.462, 53.016) centre (57.208, 53.016) ccw
  arc A2408 (56.954, 53.016) -> (57.462, 53.016) centre (57.208, 53.016) ccw
  arc A2409 (37.082, 52.6985) -> (37.082, 53.3335) centre (37.082, 53.016) ccw
  arc A2410 (36.828, 53.016) -> (37.336, 53.016) centre (37.082, 53.016) ccw
  line L3937 (53.895, 46.3495) -> (53.895, 48.6225)
  arc A2411 (37.082, 53.143) -> (37.082, 52.889) centre (37.082, 53.016) ccw
  arc A2412 (37.082, 52.6985) -> (37.082, 53.3335) centre (37.082, 53.016) ccw
  arc A2413 (36.828, 53.016) -> (37.336, 53.016) centre (37.082, 53.016) ccw
  line L3938 (56.954, 53.016) -> (57.462, 53.016)
  line L3939 (36.828, 53.016) -> (37.336, 53.016)
  line L3940 (54.395, 52.0775) -> (54.395, 54.3505)
  line L3941 (36.828, 53.016) -> (37.336, 53.016)
  line L3942 (36.828, 53.016) -> (37.336, 53.016)
  line L3943 (53.395, 52.0775) -> (53.395, 54.3505)
  arc A2414 (37.336, 53.016) -> (36.828, 53.016) centre (37.082, 53.016) ccw
  line L3944 (37.082, 52.762) -> (37.082, 53.27)
  arc A2415 (36.828, 53.016) -> (37.336, 53.016) centre (37.082, 53.016) ccw
  line L3945 (37.082, 52.762) -> (37.082, 53.27)
  line L3946 (37.082, 52.762) -> (37.082, 53.27)
  arc A2416 (37.336, 53.016) -> (36.828, 53.016) centre (37.082, 53.016) ccw
  line L3947 (53.395, 46.3495) -> (53.395, 48.6225)
  line L3948 (57.208, 52.762) -> (57.208, 53.27)
  line L3949 (54.395, 46.3495) -> (54.395, 48.6225)
  arc A2417 (36.828, 53.016) -> (37.336, 53.016) centre (37.082, 53.016) ccw
  arc A2418 (56.954, 53.016) -> (57.462, 53.016) centre (57.208, 53.016) ccw
  line L3950 (36.828, 53.016) -> (37.336, 53.016)
  arc A2419 (36.828, 53.016) -> (37.336, 53.016) centre (37.082, 53.016) ccw
  line L3951 (37.082, 52.762) -> (37.082, 53.27)
  arc A2420 (37.336, 53.016) -> (36.828, 53.016) centre (37.082, 53.016) ccw
  arc A2421 (37.336, 53.016) -> (36.828, 53.016) centre (37.082, 53.016) ccw
  line L3952 (56.954, 53.016) -> (57.462, 53.016)
  line L3953 (39.643, 58.535) -> (39.643, 58.085)
  line L3954 (39.243, 58.535) -> (39.243, 58.085)
  arc A2422 (38.143, 56.9842) -> (38.143, 57.0858) centre (38.143, 57.035) ccw
  arc A2423 (57.462, 53.016) -> (56.954, 53.016) centre (57.208, 53.016) ccw
  arc A2424 (40.1329, 58.8806) -> (39.9019, 58.8806) centre (40.0174, 58.8806) ccw
  arc A2425 (39.9019, 58.8806) -> (40.1329, 58.8806) centre (40.0174, 58.8806) ccw
  arc A2426 (57.208, 52.6985) -> (57.208, 53.3335) centre (57.208, 53.016) ccw
  line L3955 (56.954, 53.016) -> (57.462, 53.016)
  arc A2427 (40.343, 58.4842) -> (40.343, 58.5858) centre (40.343, 58.535) ccw
  line L3956 (56.954, 53.016) -> (57.462, 53.016)
  arc A2428 (37.082, 53.3335) -> (37.082, 52.6985) centre (37.082, 53.016) ccw
  line L3957 (36.828, 53.016) -> (37.336, 53.016)
  line L3958 (40.343, 58.535) -> (38.143, 58.535)
  arc A2429 (38.143, 57.0858) -> (38.143, 56.9842) centre (38.143, 57.035) ccw
  line L3959 (57.208, 52.762) -> (57.208, 53.27)
  arc A2430 (56.954, 53.016) -> (57.462, 53.016) centre (57.208, 53.016) ccw
  line L3960 (57.208, 52.762) -> (57.208, 53.27)
  line L3961 (38.143, 57.035) -> (40.343, 57.035)
  arc A2431 (37.082, 52.889) -> (37.082, 53.143) centre (37.082, 53.016) ccw
  arc A2432 (56.954, 53.016) -> (57.462, 53.016) centre (57.208, 53.016) ccw
  line L3962 (57.208, 52.762) -> (57.208, 53.27)
  line L3963 (57.208, 52.762) -> (57.208, 53.27)
  line L3964 (36.828, 53.016) -> (37.336, 53.016)
  arc A2433 (56.954, 53.016) -> (57.462, 53.016) centre (57.208, 53.016) ccw
  arc A2434 (57.208, 53.143) -> (57.208, 52.889) centre (57.208, 53.016) ccw
  arc A2435 (56.954, 53.016) -> (57.462, 53.016) centre (57.208, 53.016) ccw
  line L3965 (39.643, 58.535) -> (39.643, 58.085)
  line L3966 (40.343, 57.035) -> (40.343, 58.535)
  line L3967 (56.954, 53.016) -> (57.462, 53.016)
  line L3968 (36.828, 53.016) -> (37.336, 53.016)
  line L3969 (39.643, 58.535) -> (39.643, 58.085)
  arc A2436 (57.462, 53.016) -> (56.954, 53.016) centre (57.208, 53.016) ccw
  line L3970 (38.843, 58.535) -> (38.843, 58.085)
  arc A2437 (57.208, 52.889) -> (57.208, 53.143) centre (57.208, 53.016) ccw
  arc A2438 (36.828, 53.016) -> (37.336, 53.016) centre (37.082, 53.016) ccw
  arc A2439 (57.208, 52.889) -> (57.208, 53.143) centre (57.208, 53.016) ccw
  arc A2440 (56.954, 53.016) -> (57.462, 53.016) centre (57.208, 53.016) ccw
  arc A2441 (57.208, 53.3335) -> (57.208, 52.6985) centre (57.208, 53.016) ccw
  line L3971 (37.082, 52.762) -> (37.082, 53.27)
  arc A2442 (37.082, 53.143) -> (37.082, 52.889) centre (37.082, 53.016) ccw
  arc A2443 (57.462, 53.016) -> (56.954, 53.016) centre (57.208, 53.016) ccw
  arc A2444 (57.462, 53.016) -> (56.954, 53.016) centre (57.208, 53.016) ccw
  arc A2445 (57.462, 53.016) -> (56.954, 53.016) centre (57.208, 53.016) ccw
  line L3972 (56.954, 53.016) -> (57.462, 53.016)
  line L3973 (57.208, 52.762) -> (57.208, 53.27)
  arc A2446 (56.954, 53.016) -> (57.462, 53.016) centre (57.208, 53.016) ccw
  arc A2447 (37.336, 53.016) -> (36.828, 53.016) centre (37.082, 53.016) ccw
  arc A2448 (36.828, 53.016) -> (37.336, 53.016) centre (37.082, 53.016) ccw
  line L3974 (57.208, 52.762) -> (57.208, 53.27)
  arc A2449 (57.462, 53.016) -> (56.954, 53.016) centre (57.208, 53.016) ccw
  arc A2450 (37.082, 52.889) -> (37.082, 53.143) centre (37.082, 53.016) ccw
  line L3975 (56.954, 53.016) -> (57.462, 53.016)
  arc A2451 (37.082, 53.143) -> (37.082, 52.889) centre (37.082, 53.016) ccw
  arc A2452 (40.343, 57.0858) -> (40.343, 56.9842) centre (40.343, 57.035) ccw
  arc A2453 (57.208, 52.6985) -> (57.208, 53.3335) centre (57.208, 53.016) ccw
  line L3976 (39.243, 58.535) -> (39.243, 58.085)
  arc A2454 (37.082, 52.889) -> (37.082, 53.143) centre (37.082, 53.016) ccw
  arc A2455 (40.343, 58.5858) -> (40.343, 58.4842) centre (40.343, 58.535) ccw
  arc A2456 (57.208, 53.143) -> (57.208, 52.889) centre (57.208, 53.016) ccw
  line L3977 (38.843, 58.535) -> (38.843, 58.085)
  arc A2457 (38.143, 58.5858) -> (38.143, 58.4842) centre (38.143, 58.535) ccw
  arc A2458 (57.462, 53.016) -> (56.954, 53.016) centre (57.208, 53.016) ccw
  line L3978 (56.954, 53.016) -> (57.462, 53.016)
  line L3979 (15.8086, 7.198) -> (15.1286, 7.198)
  line L3980 (15.391, 7.723) -> (15.391, 4.723)
  line L3981 (18.6534, 5.898) -> (17.9734, 5.898)
  line L3982 (17.691, 7.323) -> (17.091, 7.323)
  line L3983 (39.243, 57.485) -> (39.243, 57.035)
  line L3984 (38.093, 58.185) -> (38.543, 58.185)
  line L3985 (38.843, 58.535) -> (38.843, 58.085)
  line L3986 (16.091, 5.023) -> (16.691, 5.023)
  line L3987 (18.6534, 7.198) -> (17.9734, 7.198)
  line L3988 (16.691, 6.023) -> (16.091, 6.023)
  line L3989 (39.243, 58.535) -> (39.243, 58.085)
  line L3990 (39.943, 57.385) -> (40.393, 57.385)
  line L3991 (39.643, 57.485) -> (39.643, 57.035)
  line L3992 (16.091, 7.323) -> (16.091, 6.323)
  line L3993 (18.6534, 6.548) -> (17.9734, 6.548)
  line L3994 (39.943, 57.785) -> (40.393, 57.785)
  line L3995 (38.093, 57.385) -> (38.543, 57.385)
  line L3996 (18.6534, 5.248) -> (17.9734, 5.248)
  line L3997 (38.843, 57.485) -> (38.843, 57.035)
  line L3998 (17.091, 7.323) -> (17.091, 6.323)
  line L3999 (18.391, 7.723) -> (15.391, 7.723)
  arc A2459 (57.208, 53.143) -> (57.208, 52.889) centre (57.208, 53.016) ccw
  line L4000 (39.943, 58.185) -> (40.393, 58.185)
  arc A2460 (38.143, 58.4842) -> (38.143, 58.5858) centre (38.143, 58.535) ccw
  arc A2461 (19.1372, 5.0982) -> (18.7372, 5.0982) centre (18.9372, 5.0982) ccw
  line L4001 (16.091, 6.323) -> (16.691, 6.323)
  line L4002 (16.691, 6.323) -> (16.691, 7.323)
  line L4003 (15.391, 4.723) -> (18.391, 4.723)
  line L4004 (15.8086, 7.198) -> (15.1286, 7.198)
  line L4005 (15.8086, 7.198) -> (15.1286, 7.198)
  line L4006 (17.091, 5.023) -> (17.691, 5.023)
  line L4007 (38.143, 58.535) -> (38.143, 57.035)
  arc A2462 (18.7372, 5.0982) -> (19.1372, 5.0982) centre (18.9372, 5.0982) ccw
  line L4008 (18.6534, 7.198) -> (17.9734, 7.198)
  line L4009 (17.691, 6.023) -> (17.091, 6.023)
  line L4010 (39.643, 57.485) -> (39.643, 57.035)
  line L4011 (38.093, 57.785) -> (38.543, 57.785)
  line L4012 (38.843, 57.485) -> (38.843, 57.035)
  line L4013 (18.391, 4.723) -> (18.391, 7.723)
  line L4014 (39.243, 57.485) -> (39.243, 57.035)
  line L4015 (39.943, 58.185) -> (40.393, 58.185)
  line L4016 (39.643, 57.485) -> (39.643, 57.035)
  arc A2463 (57.208, 52.889) -> (57.208, 53.143) centre (57.208, 53.016) ccw
  line L4017 (39.943, 57.785) -> (40.393, 57.785)
  line L4018 (57.208, 52.762) -> (57.208, 53.27)
  arc A2464 (57.208, 53.3335) -> (57.208, 52.6985) centre (57.208, 53.016) ccw
  line L4019 (38.093, 58.185) -> (38.543, 58.185)
  line L4020 (57.208, 52.762) -> (57.208, 53.27)
  arc A2465 (56.954, 53.016) -> (57.462, 53.016) centre (57.208, 53.016) ccw
  line L4021 (38.093, 58.185) -> (38.543, 58.185)
  line L4022 (38.093, 57.385) -> (38.543, 57.385)
  arc A2466 (57.462, 53.016) -> (56.954, 53.016) centre (57.208, 53.016) ccw
  line L4023 (56.954, 53.016) -> (57.462, 53.016)
  line L4024 (56.954, 53.016) -> (57.462, 53.016)
  arc A2467 (40.343, 56.9842) -> (40.343, 57.0858) centre (40.343, 57.035) ccw
  line L4025 (39.943, 57.785) -> (40.393, 57.785)
  line L4026 (38.093, 57.785) -> (38.543, 57.785)
  line L4027 (39.943, 57.385) -> (40.393, 57.385)
  line L4028 (38.093, 57.785) -> (38.543, 57.785)
  line L4029 (38.843, 57.485) -> (38.843, 57.035)
  line L4030 (39.243, 57.485) -> (39.243, 57.035)
  line L4031 (38.093, 57.385) -> (38.543, 57.385)
  line L4032 (39.943, 57.385) -> (40.393, 57.385)
  line L4033 (18.6534, 5.248) -> (17.9734, 5.248)
  arc A2468 (71.6788, 9.906) -> (69.4436, 9.906) centre (70.5612, 9.906) ccw
  line L4034 (70.3072, 9.906) -> (70.8152, 9.906)
  arc A2469 (69.4436, 9.906) -> (71.6788, 9.906) centre (70.5612, 9.906) ccw
  line L4035 (69.281, 55.14) -> (69.281, 53.74)
  arc A2470 (69.4436, 9.906) -> (71.6788, 9.906) centre (70.5612, 9.906) ccw
  line L4036 (39.943, 58.185) -> (40.393, 58.185)
  line L4037 (92.71, 30.4546) -> (93.726, 30.4546)
  line L4038 (15.8086, 5.248) -> (15.1286, 5.248)
  arc A2471 (70.8914, 9.906) -> (70.231, 9.906) centre (70.5612, 9.906) ccw
  line L4039 (70.5612, 9.652) -> (70.5612, 10.16)
  line L4040 (16.091, 6.023) -> (16.091, 5.023)
  line L4041 (15.8086, 5.248) -> (15.1286, 5.248)
  line L4042 (18.6534, 5.898) -> (17.9734, 5.898)
  line L4043 (91.948, 30.226) -> (91.948, 28.321)
  line L4044 (68.981, 54.94) -> (68.981, 51.74)
  line L4045 (17.091, 6.323) -> (17.691, 6.323)
  line L4046 (15.8086, 5.248) -> (15.1286, 5.248)
  line L4047 (92.583, 27.686) -> (94.488, 27.686)
  line L4048 (92.71, 27.4574) -> (93.726, 27.4574)
  line L4049 (94.7166, 27.8511) -> (94.7166, 30.0609)
  line L4050 (92.71, 27.4574) -> (93.726, 27.4574)
  line L4051 (94.7166, 27.8511) -> (94.7166, 30.0609)
  line L4052 (15.8086, 5.898) -> (15.1286, 5.898)
  line L4053 (91.7194, 27.8511) -> (91.7194, 30.0609)
  line L4054 (15.8086, 6.548) -> (15.1286, 6.548)
  line L4055 (92.2274, 27.9654) -> (94.2086, 27.9654)
  line L4056 (15.8086, 6.548) -> (15.1286, 6.548)
  arc A2472 (70.231, 9.906) -> (70.8914, 9.906) centre (70.5612, 9.906) ccw
  line L4057 (16.691, 5.023) -> (16.691, 6.023)
  line L4058 (70.3072, 9.906) -> (70.8152, 9.906)
  line L4059 (94.2086, 27.9654) -> (94.2086, 29.9466)
  line L4060 (16.691, 7.323) -> (16.091, 7.323)
  line L4061 (91.7194, 27.8511) -> (91.7194, 30.0609)
  line L4062 (71.481, 54.94) -> (68.981, 54.94)
  line L4063 (70.5612, 9.652) -> (70.5612, 10.16)
  line L4064 (92.71, 27.4574) -> (93.726, 27.4574)
  arc A2473 (70.8914, 9.906) -> (70.231, 9.906) centre (70.5612, 9.906) ccw
  line L4065 (69.281, 52.94) -> (69.281, 51.54)
  line L4066 (16.891, 5.033) -> (16.891, 7.413)
  line L4067 (16.891, 5.033) -> (16.891, 7.413)
  line L4068 (15.8086, 6.548) -> (15.1286, 6.548)
  line L4069 (18.6534, 7.198) -> (17.9734, 7.198)
  line L4070 (15.8086, 5.898) -> (15.1286, 5.898)
  line L4071 (94.488, 30.226) -> (91.948, 30.226)
  line L4072 (18.6534, 5.898) -> (17.9734, 5.898)
  line L4073 (18.6534, 5.248) -> (17.9734, 5.248)
  line L4074 (18.6534, 6.548) -> (17.9734, 6.548)
  line L4075 (94.7166, 27.8511) -> (94.7166, 30.0609)
  line L4076 (92.2274, 29.9466) -> (92.2274, 27.9654)
  line L4077 (94.2086, 29.9466) -> (92.2274, 29.9466)
  line L4078 (17.691, 6.323) -> (17.691, 7.323)
  line L4079 (91.948, 28.321) -> (92.583, 27.686)
  line L4080 (17.691, 5.023) -> (17.691, 6.023)
  line L4081 (92.71, 30.4546) -> (93.726, 30.4546)
  line L4082 (91.7194, 27.8511) -> (91.7194, 30.0609)
  line L4083 (15.8086, 5.898) -> (15.1286, 5.898)
  line L4084 (18.6534, 6.548) -> (17.9734, 6.548)
  line L4085 (68.981, 51.74) -> (71.481, 51.74)
  line L4086 (92.71, 30.4546) -> (93.726, 30.4546)
  line L4087 (94.488, 27.686) -> (94.488, 30.226)
  arc A2474 (72.331, 51.9238) -> (72.331, 52.5562) centre (72.331, 52.24) ccw
  arc A2475 (71.6788, 9.906) -> (69.4436, 9.906) centre (70.5612, 9.906) ccw
  arc A2476 (70.231, 9.906) -> (70.8914, 9.906) centre (70.5612, 9.906) ccw
  line L4088 (17.091, 6.023) -> (17.091, 5.023)
  line L4089 (71.481, 51.74) -> (71.481, 54.94)
  arc A2477 (69.4436, 9.906) -> (71.6788, 9.906) centre (70.5612, 9.906) ccw
  arc A2478 (70.5612, 9.3472) -> (70.5612, 10.4648) centre (70.5612, 9.906) ccw
  line L4090 (70.5612, 9.652) -> (70.5612, 10.16)
  arc A2479 (70.5612, 10.4648) -> (70.5612, 9.3472) centre (70.5612, 9.906) ccw
  arc A2480 (70.5612, 9.3472) -> (70.5612, 10.4648) centre (70.5612, 9.906) ccw
  arc A2481 (70.8914, 9.906) -> (70.231, 9.906) centre (70.5612, 9.906) ccw
  line L4091 (83.2612, 9.525) -> (83.2612, 10.033)
  arc A2482 (82.931, 9.779) -> (83.5914, 9.779) centre (83.2612, 9.779) ccw
  line L4092 (71.181, 55.14) -> (71.181, 53.74)
  arc A2483 (82.931, 9.779) -> (83.5914, 9.779) centre (83.2612, 9.779) ccw
  arc A2484 (82.931, 9.779) -> (83.5914, 9.779) centre (83.2612, 9.779) ccw
  line L4093 (69.281, 55.14) -> (69.281, 53.74)
  line L4094 (83.0072, 9.779) -> (83.5152, 9.779)
  arc A2485 (82.931, 9.779) -> (83.5914, 9.779) centre (83.2612, 9.779) ccw
  line L4095 (70.5612, 9.652) -> (70.5612, 10.16)
  line L4096 (69.281, 52.94) -> (69.281, 51.54)
  line L4097 (83.2612, 9.525) -> (83.2612, 10.033)
  arc A2486 (70.8914, 9.906) -> (70.231, 9.906) centre (70.5612, 9.906) ccw
  arc A2487 (70.231, 9.906) -> (70.8914, 9.906) centre (70.5612, 9.906) ccw
  line L4098 (83.2612, 9.525) -> (83.2612, 10.033)
  arc A2488 (70.5612, 10.4648) -> (70.5612, 9.3472) centre (70.5612, 9.906) ccw